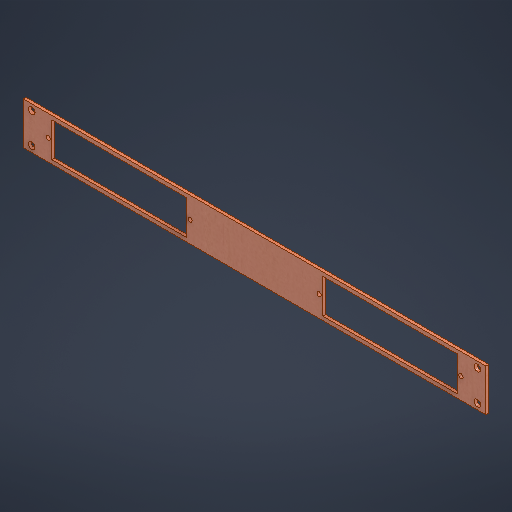
# Autodesk Inventor part: WoodPanel
Saved by Autodesk Inventor 2026.2 (Build 302298010, 298A)
## iProperties
Created: 2026-03-25
Part Number: WoodPanel
Material: Wood (Walnut)
Document SubType Name: Modeling
Designer: usr
Density: 0.55 g/cm^3
Appearance: Walnut - Natural Polished
Author: usr
Autodesk Inventor part; units mm, degrees
ref_plane "YZ Plane" through (0, 0, 0) normal (1, 0, 0) x (0, 1, 0)
ref_plane "XZ Plane" through (0, 0, 0) normal (0, 1, 0) x (-1, 0, 0)
ref_plane "XY Plane" through (0, 0, 0) normal (0, 0, 1) x (1, 0, 0)
sketch "Sketch1" plane through (0, 0, 0) normal (0, 0, 1) x (1, 0, 0)
  line L0 (0, 0) -> (-482.6, 0)
  line L1 (-482.6, 0) -> (-482.6, 44)
  line L2 (-482.6, 44) -> (0, 44)
  line L3 (0, 44) -> (0, 0)
  circle A0 centre (-473.8, 37.875) radius 3.5
  circle A1 centre (-473.8, 6.125) radius 3.5
  circle A2 centre (-8.8, 37.875) radius 3.5
  circle A3 centre (-8.8, 6.125) radius 3.5
  dimension "d0" = 44
  dimension "d1" = 482.6
  dimension "d5" = 31.75
  dimension "d6" = 7
  dimension "d8" = 31.75
  dimension "d9" = 465
  dimension "d10" = 465
  dimension "d11" = 8.8
  dimension "d12" = 8.8
  dimension "d13" = 6.125
  dimension "d14" = 6.125
  dimension "d15" = 6.125
  dimension "d16" = 8.8
  dimension "d17" = 8.8
  dimension "d18" = 6.125
  constraints: 8 end point, 4 centre point, 3 equal radius, 2 parallel, 1 horizontal, 1 perpendicular
  measures "d0" distance between parallel lines of L0 L2
  measures "d1" distance between parallel lines of L1 L3
  measures "d5" distance of A1.centre A0.centre
  measures "d6" diameter of A2
  measures "d8" distance of A2.centre A3.centre
  measures "d9" distance of A1.centre A3.centre
  measures "d10" distance of A2.centre A0.centre
  measures "d11" distance from line of L3 A3.centre
  measures "d12" distance from line of L3 A2.centre
  measures "d13" distance from line of L2 A2.centre
  measures "d14" distance from line of L0 A3.centre
  measures "d15" distance from line of L2 A0.centre
  measures "d16" distance from line of L1 A1.centre
  measures "d17" distance from line of L1 A0.centre
  measures "d18" distance from line of L0 A1.centre
extrude "Frame" add sketch "Sketch1" along normal blind 3
sketch "Sketch2" plane through (0, 0, 3) normal (0, 0, 1) x (1, 0, 0)
  line L0 (-30, 4) -> (-170, 4)
  line L1 (-170, 4) -> (-170, 40)
  line L2 (-170, 40) -> (-30, 40)
  line L3 (-30, 40) -> (-30, 4)
  line L4 (-452.6003, 40) -> (-312.6003, 40)
  line L5 (-312.6003, 40) -> (-312.6003, 4)
  line L6 (-312.6003, 4) -> (-452.6003, 4)
  line L7 (-452.6003, 4) -> (-452.6003, 40)
  line L8 (0, 0) -> (0, 44) projected
  line L9 (0, 44) -> (-482.6, 44) projected
  line L10 (-482.6, 44) -> (-482.6, 0) projected
  point P0 (-30, 22)
  point P1 (-312.6003, 22)
  dimension "d21" = 140
  dimension "d22" = 36
  dimension "d25" = 30
  dimension "d26" = 22
  dimension "d27" = 22
  dimension "d28" = 29.9997
  constraints: 16 end point, 4 parallel, 2 equal length, 2 horizontal, 2 midpoint, 2 perpendicular
  measures "d21" distance of L1.end L2.end
  measures "d22" distance of L0.end L1.end
  measures "d25" distance between parallel lines of L8 L3
  measures "d26" distance from line of point (-30, 22) L9
  measures "d27" distance from line of point (-312.6, 22) L9
  measures "d28" distance between parallel lines of L10 L7
extrude "PI_Holes" cut sketch "Sketch2" against normal blind 5
sketch "Sketch4" plane through (0, 0, 3) normal (0, 0, 1) x (1, 0, 0)
  circle A0 centre (-26, 22) radius 2 projected
  circle A1 centre (-174, 22) radius 2 projected
  circle A2 centre (-308.6003, 22) radius 2 projected
  circle A3 centre (-456.6003, 22) radius 2 projected
  circle A4 centre (-456.6003, 22) radius 2.25
  circle A5 centre (-308.6003, 22) radius 2.25
  circle A6 centre (-174, 22) radius 2.25
  circle A7 centre (-26, 22) radius 2.25
  point P0 (0, 0)
  dimension "d35" = 4
  dimension "d36" = 4.5
  dimension "d37" = 4.5
  dimension "d38" = 4.5
  dimension "d39" = 4.5
  constraints: 4 centre point, 4 coincident
  measures "d35" diameter of A2
  measures "d36" diameter of A4
  measures "d37" diameter of A5
  measures "d38" diameter of A6
  measures "d39" diameter of A7
extrude "Mounting_Holes" cut sketch "Sketch4" against normal through all contours A0 | A1 | A2 | A3 | A4 | A5 | A6 | A7
body "Solid1"
